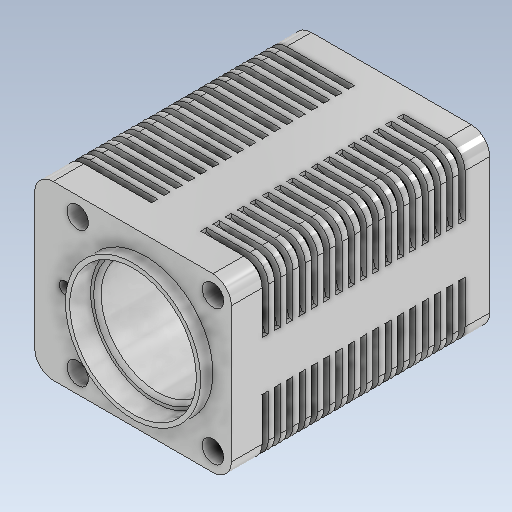
# Autodesk Inventor part: Peça6
Saved by Autodesk Inventor 2021 (Build 250183000, 183)
## iProperties
Category: 42
Created: 2021-07-18
Part Number: Peça6
Material: Alumínio 6061
Document SubType Name: Modeling
Designer: Giovanni
Density: 2.7 g/cm^3
Appearance: Alumínio - Polido
User Status: 1:4
Author: Giovanni
Keywords: 10
Autodesk Inventor part; units mm, degrees
ref_plane "YZ Plane" through (0, 0, 0) normal (1, 0, 0) x (0, 1, 0)
ref_plane "XZ Plane" through (0, 0, 0) normal (0, 1, 0) x (-1, 0, 0)
sketch "Esboço1" plane through (0, 0, 0) normal (0, 0, 1) x (1, 0, 0)
  line L0 (-75, 70) -> (55, 70)
  line L1 (70, 55) -> (70, -55)
  line L2 (55, -70) -> (-75, -70)
  line L3 (-90, -55) -> (-90, 55)
  arc A0 (-75, 70) -> (-90, 55) centre (-75, 55) ccw
  arc A1 (70, 55) -> (55, 70) centre (55, 55) ccw
  arc A2 (55, -70) -> (70, -55) centre (55, -55) ccw
  arc A3 (-90, -55) -> (-75, -70) centre (-75, -55) ccw
  point P0 (0, 0)
  point P1 (70, -70)
  point P2 (70, 70)
  point P3 (-90, -70)
  point P4 (70, 0)
  dimension "d0" = 140
  dimension "d1" = 160
  dimension "d2" = 70
  dimension "d3" = 15
  constraints: 8 end point, 8 point on circle, 8 tangent, 6 point on line, 4 centre point, 3 equal radius, 2 parallel, 1 horizontal, 1 horizontal alignment, 1 midpoint, 1 perpendicular
  measures "d0" distance of point (70, 70) point (70, -70)
  measures "d1" distance of point (70, -70) point (-90, -70)
  measures "d2" distance from line of L1 point (0, 0)
  measures "d3" radius of A0
extrude "Extrusão1" add sketch "Esboço1" along normal blind 210
sketch "Esboço2" plane through (0, 0, 210) normal (0, 0, -1) x (-1, 0, 0)
  circle A0 centre (0, 0) radius 55
  dimension "d6" = 110
  constraints: 1 centre point, 1 coincident
  measures "d6" diameter of A0
extrude "Extrusão2" add sketch "Esboço2" against normal blind 10
sketch "Esboço3" plane through (0, 0, 220) normal (0, 0, 1) x (1, 0, 0)
  circle A0 centre (0, 0) radius 51.5
  dimension "d9" = 103
  constraints: 1 centre point, 1 coincident
  measures "d9" diameter of A0
extrude "Extrusão3" cut sketch "Esboço3" against normal blind 17
ref_plane "Plano de trabalho1" through (0, 0, 20) normal (0, 0, -1) x (-1, 0, 0)
sketch "Esboço5" plane through (0, 0, 20) normal (0, 0, -1) x (-1, 0, 0)
  line L0 (67.082, 20) -> (90, 20)
  line L1 (67.082, -20) -> (90, -20)
  line L2 (-67.082, 20) -> (-70, 20)
  line L3 (-67.082, -20) -> (-70, -20)
  line L4 (-20, 67.082) -> (-20, 70)
  line L5 (20, 67.082) -> (20, 70)
  line L6 (-20, -67.082) -> (-20, -70)
  line L7 (20, -67.082) -> (20, -70)
  arc A0 (-55, 70) -> (-70, 55) centre (-55, 55) ccw projected
  line L8 (-55, 70) -> (75, 70) projected
  arc A1 (90, 55) -> (75, 70) centre (75, 55) ccw projected
  line L9 (90, 55) -> (90, -55) projected
  arc A2 (75, -70) -> (90, -55) centre (75, -55) ccw projected
  line L10 (75, -70) -> (-55, -70) projected
  arc A3 (-70, -55) -> (-55, -70) centre (-55, -55) ccw projected
  line L11 (-70, -55) -> (-70, 55) projected
  arc A4 (67.082, 20) -> (20, 67.082) centre (0, 0) ccw
  arc A5 (-20, 67.082) -> (-67.082, 20) centre (0, 0) ccw
  arc A6 (-67.082, -20) -> (-20, -67.082) centre (0, 0) ccw
  arc A7 (20, -67.082) -> (67.082, -20) centre (0, 0) ccw
  dimension "d23" = 70
  dimension "d24" = 40
  dimension "d25" = 20
  dimension "d26" = 40
  dimension "d27" = 20
  constraints: 16 end point, 8 point on circle, 8 point on line, 4 centre point, 4 collinear, 4 horizontal, 4 vertical, 3 concentric, 1 coincident
  measures "d23" radius of A5
  measures "d24" distance between parallel lines of L1 L0
  measures "d25" distance from line of point (0, 0) L0
  measures "d26" distance of L5.end L4.end
  measures "d27" horizontal distance of point (0, 0) L4.end
extrude "Extrusão4" cut sketch "Esboço5" against normal blind 5 contours A4 L5 L8 A1 L9 L0 | L9 A2 L10 L7 A7 L1 | L4 A5 L2 L11 A0 L8 | L10 A3 L11 L3 A6 L6
pattern_linear "Padrão retangular1" count 17 spacing 10 along (0, 0, 1) of "Extrusão4"
sketch "Esboço9" plane through (0, 0, 0) normal (0, 0, -1) x (-1, 0, 0)
  arc A0 (-70, -55) -> (-55, -70) centre (-55, -55) ccw projected
  arc A1 (-55, 70) -> (-70, 55) centre (-55, 55) ccw projected
  arc A2 (90, 55) -> (75, 70) centre (75, 55) ccw projected
  arc A3 (75, -70) -> (90, -55) centre (75, -55) ccw projected
  point P0 (0, 0)
  point P1 (55, 55)
  point P2 (55, -55)
  dimension "d50" = 55
  dimension "d51" = 55
  constraints: 2 coincident, 2 horizontal alignment
  measures "d50" horizontal distance of point (0, 0) point (55, -55)
  measures "d51" horizontal distance of point (0, 0) point (55, 55)
hole "Furo2" at (55, -55, 0) at (55, 55, 0) at (-55, 55, 0) at (-55, -55, 0) direction (0, 0, 1) diameter 17.5 end through all
sketch "Esboço14" plane through (0, 0, 203) normal (0, 0, 1) x (1, 0, 0)
  circle A0 centre (0, 0) radius 46
  dimension "d90" = 92
  constraints: 1 centre point, 1 coincident
  measures "d90" diameter of A0
extrude "Extrusão8" cut sketch "Esboço14" against normal through all
chamfer "Chanfro1" distance 3 angle 45 1 edges at (-46, 0, 203)
sketch "Esboço15" plane through (0, 0, 0) normal (0, 0, -1) x (-1, 0, 0)
  circle A0 centre (0, 0) radius 52.5
  dimension "d96" = 105
  constraints: 1 centre point, 1 coincident
  measures "d96" diameter of A0
extrude "Extrusão9" cut sketch "Esboço15" against normal blind 7
sketch "Esboço16" plane through (0, 0, 0) normal (0, 0, -1) x (-1, 0, 0)
  arc A0 (65, -5) -> (65, 5) centre (65, 0) ccw
  line L0 (65, -5) -> (40, -5)
  line L1 (40, -5) -> (40, 5)
  line L2 (40, 5) -> (65, 5)
  point P0 (0, 0)
  dimension "d99" = 10
  dimension "d100" = 65
  dimension "d101" = 25
  constraints: 6 end point, 2 point on circle, 1 centre point, 1 horizontal, 1 horizontal alignment, 1 perpendicular, 1 tangent
  measures "d99" diameter of A0
  measures "d100" distance of point (0, 0) A0.centre
  measures "d101" distance from line of L1 A0.centre
extrude "Extrusão10" cut sketch "Esboço16" against normal blind 10
sketch "Esboço17" plane through (0, 0, 10) normal (0, 0, -1) x (-1, 0, 0)
  arc A0 (65, -5) -> (65, 5) centre (65, 0) ccw projected
  point P0 (0, 0)
  constraints: 1 coincident
hole "Furo6" at (-65, 0, 10) direction (0, 0, 1) diameter 10 end through all
